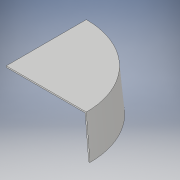
# Autodesk Inventor part: QuarterTop
Saved by Autodesk Inventor 2019 (Build 230136000, 136)
## iProperties
Created: 2019-10-09
Part Number: QuarterTop
Material: Generic
Document SubType Name: Modeling
Designer: james
Density: 1 g/cm^3
Appearance: Default
Author: james
Autodesk Inventor part; units mm, degrees
ref_plane "YZ Plane" through (0, 0, 0) normal (1, 0, 0) x (0, 1, 0)
ref_plane "XZ Plane" through (0, 0, 0) normal (0, 1, 0) x (-1, 0, 0)
ref_plane "XY Plane" through (0, 0, 0) normal (0, 0, 1) x (1, 0, 0)
sketch "Sketch1" plane through (0, 0, 0) normal (1, 0, 0) x (0, 1, 0)
  line L0 (52.2781, 123.0082) -> (49.1031, 123.0082)
  line L1 (-49.3219, -80.1918) -> (-49.3219, -77.0168)
  line L2 (-49.3219, -77.0168) -> (49.1031, -68.4058)
  line L3 (52.2781, -68.128) -> (52.2781, -71.303)
  line L4 (-49.3219, -80.1918) -> (52.2781, -71.303)
  line L5 (52.2781, -68.128) -> (52.2781, 123.0082)
  line L6 (49.1031, 123.0082) -> (49.1031, -68.4058)
  point P0 (0, 0)
  dimension "d0" = 203.2
  dimension "d1" = 3.175
  dimension "d2" = 95
  dimension "d3" = 101.6
  dimension "d4" = 180
  dimension "d5" = 3.175
  constraints: 14 end point, 3 vertical, 1 horizontal, 1 parallel
  measures "d0" distance from line of L0 L1.start
  measures "d1" distance of L1.start L1.end
  measures "d2" angle of L2 L1
  measures "d3" distance between parallel lines of L1 L3
  measures "d4" angle of L2 L4
  measures "d5" distance between parallel lines of L6 L5
revolve "Revolution1" add sketch "Sketch1" angle 90 about axis through (0, 52.2781, 123.0082) along (0, -1, 0)
body "Solid1"
